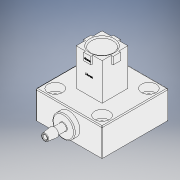
# Autodesk Inventor part: 9mm_ball_holder
Saved by Autodesk Inventor 2019 (Build 230136000, 136)
## iProperties
Created: 2019-03-11
Part Number: 9mm_ball_holder
Material: ABS Plastic
Document SubType Name: Modeling
Designer: Wilson Lab
Density: 1.06 g/cm^3
Appearance: Smooth - White
Author: Wilson Lab
Autodesk Inventor part; units mm, degrees
ref_plane "YZ Plane" through (0, 0, 0) normal (1, 0, 0) x (0, 1, 0)
ref_plane "XZ Plane" through (0, 0, 0) normal (0, 1, 0) x (-1, 0, 0)
ref_plane "XY Plane" through (0, 0, 0) normal (0, 0, 1) x (1, 0, 0)
sketch "Sketch1" plane through (0, 0, 0) normal (0, 0, 1) x (1, 0, 0)
  line L0 (0, 0) -> (-7, 0) construction
  line L1 (-7, 0) -> (-7, 20) construction
  line L2 (-7, 20) -> (0, 20) construction
  line L3 (0, 20) -> (0, 0) construction
  circle A0 centre (0, 20.35) radius 6 construction
  line L4 (-7, 20) -> (-6.6598, 20)
  line L5 (-0.75, 13.7688) -> (-0.75, 0)
  arc A1 (-5.9198, 19.3722) -> (-1.3333, 14.5) centre (0, 20.35) ccw
  arc A2 (-0.75, 13.7688) -> (-1.3333, 14.5) centre (-1.5, 13.7688) ccw
  arc A3 (-5.9198, 19.3722) -> (-6.6598, 20) centre (-6.6598, 19.25) ccw
  line L6 (-7, 20) -> (-7, 0)
  line L7 (-7, 0) -> (-0.75, 0)
  point P0 (-5.9898, 20)
  point P1 (-0.75, 14.3971)
  dimension "d0" = 7
  dimension "d1" = 20
  dimension "d5" = 12
  dimension "d6" = 0.35
  dimension "d7" = 0.75
  dimension "d8" = 0.75
  dimension "d9" = 0.75
  dimension "d132" = 1.0102
  constraints: 18 end point, 10 point on circle, 5 point on line, 4 centre point, 4 tangent, 3 perpendicular, 2 parallel, 1 collinear, 1 concentric, 1 horizontal
  measures "d0" distance between parallel lines of L3 L1
  measures "d1" distance between parallel lines of L0 L2
  measures "d5" diameter of A0
  measures "d6" distance of A0.centre L2.end
  measures "d7" distance between parallel lines of L3 L5
  measures "d8" radius of A2
  measures "d9" radius of A3
  measures "d132" distance of A0.start L1.end
revolve "Revolution1" add sketch "Sketch1" angle 360 about axis through (0, 20, 0) along (0, -1, 0)
ref_plane "Work Plane1" through (0, 20, 0) normal (0, 1, 0) x (1, 0, 0)
sketch "Sketch2" plane through (0, 20, 0) normal (0, 1, 0) x (1, 0, 0)
  circle A0 centre (0, 0) radius 7 projected
  circle A1 centre (0, 0) radius 7 construction
  line L0 (-7, -7) -> (7, -7)
  line L1 (7, -7) -> (7, 7)
  line L2 (7, 7) -> (-7, 7)
  line L3 (-7, 7) -> (-7, -7)
  circle A2 centre (0, 0) radius 1.3333 projected
  line L4 (-7, -7) -> (7, 7) construction
  line L5 (7, -7) -> (-7, 7) construction
  point P0 (0, 0)
  dimension "d124" = 0
  constraints: 12 end point, 2 midpoint, 2 parallel, 2 tangent, 1 centre point, 1 coincident, 1 horizontal, 1 perpendicular
  measures "d124" distance edge to line of A0 L1
extrude "Extrusion1" add sketch "Sketch2" against normal up to surface (20 mm away) contours L1 L0 A0 | A0 L2 L1 | A0 L3 L2 | L0 L3 A0
ref_plane "Work Plane7" through (0, 0, 0) normal (0, -1, 0) x (1, 0, 0)
sketch "Sketch11" plane through (0, 0, 0) normal (0, -1, 0) x (1, 0, 0)
  line L0 (0, 18) -> (0, 0) construction
  line L1 (-18, -18) -> (18, -18)
  line L2 (18, -18) -> (18, 18)
  line L3 (18, 18) -> (-18, 18)
  line L4 (-18, 18) -> (-18, -18)
  line L5 (-18, -18) -> (18, 18) construction
  line L6 (18, -18) -> (-18, 18) construction
  dimension "d60" = 36
  dimension "d61" = 36
  constraints: 14 end point, 3 midpoint, 2 parallel, 1 horizontal, 1 perpendicular
  measures "d60" distance of L1.end L2.end
  measures "d61" distance of L2.end L3.end
extrude "Extrusion6" add sketch "Sketch11" along normal blind 15
sketch "Sketch16" plane through (-18, 0, -18) normal (-1, 0, 0) x (0, 0, 1)
  line L0 (36, 0) -> (0, 0) construction
  line L1 (0, 0) -> (0, -15) construction
  line L2 (36, -15) -> (0, -15) construction
  line L3 (36, 0) -> (36, -15) construction
  line L4 (18.75, 13.7688) -> (18.75, 0) construction
  line L5 (17.25, 13.7688) -> (17.25, 0) construction
  line L6 (18, -7.5) -> (18, 0) construction
  line L7 (36, 0) -> (36, -15) construction
  line L8 (36, 0) -> (36, -7.5) construction
  line L9 (18, -7.5) -> (36, -7.5) construction
  circle A0 centre (18, -7.5) radius 4.225
  dimension "d64" = 8.45
  constraints: 6 end point, 1 centre point, 1 coincident, 1 horizontal, 1 midpoint, 1 vertical
  measures "d64" diameter of A0
extrude "Extrusion7" cut sketch "Sketch16" against normal blind 32.7
sketch "Sketch17" plane through (0, 0, 0) normal (0, -1, 0) x (1, 0, 0)
  circle A0 centre (0, 0) radius 0.75 projected
  point P0 (0, 0)
ref_plane "Work Plane8" through (-18, 0, 0) normal (0, 0, 1) x (1, 0, 0)
sketch "Sketch18" plane through (-18, 0, 0) normal (0, 0, 1) x (1, 0, 0)
  line L0 (18, 0) -> (18, -10.576)
  line L1 (0, -11.725) -> (32.7, -11.725) projected
  constraints: 2 end point, 1 vertical
sweep "Sweep3" cut profiles "Sketch17" path "Sketch18" path curves L0
fillet "Fillet1" radius 3 1 edges at (-0.75, -3.275, -0.001)
sketch "Sketch19" plane through (0, 0, 0) normal (0, 1, 0) x (1, 0, 0)
  line L0 (18, -18) -> (-18, -18) construction
  line L1 (18, 18) -> (18, -18) construction
  line L2 (-18, 18) -> (18, 18) construction
  line L3 (-18, -18) -> (-18, 18) construction
  line L4 (-12.7, 12.7) -> (12.7, 12.7) construction
  line L5 (12.7, 12.7) -> (12.7, -12.7) construction
  line L6 (12.7, -12.7) -> (-12.7, -12.7) construction
  line L7 (-12.7, -12.7) -> (-12.7, 12.7) construction
  circle A0 centre (0, 0) radius 1.3333 construction
  line L8 (-12.7, 12.7) -> (12.7, -12.7) construction
  line L9 (12.7, 12.7) -> (-12.7, -12.7) construction
  point P0 (0, 0)
  dimension "d70" = 25.4
  dimension "d71" = 25.4
  constraints: 12 end point, 4 coincident, 2 midpoint, 2 parallel, 1 horizontal, 1 perpendicular
  measures "d70" distance of L4.end L5.end
  measures "d71" distance of L5.end L6.end
hole "Hole3" at (12.7, 0, -12.7) at (12.7, 0, 12.7) at (-12.7, 0, 12.7) at (-12.7, 0, -12.7) direction (0, -1, 0) diameter 4.496 end through all counterbore diameter 7.938 counterbore depth 4.166
sketch "Sketch21" plane through (-18, 0, 0) normal (0, 0, 1) x (1, 0, 0)
  line L0 (0, -11.725) -> (0, -3.275) construction
  line L1 (0, 0) -> (0, -15) construction
  line L2 (0, -7.5) -> (-3, -7.5)
  line L3 (-3, -9.6296) -> (-3, -13.5)
  line L4 (-3, -13.5) -> (0, -13.5)
  line L5 (0, -13.5) -> (0, -7.5) construction
  line L6 (-3.25, -9.3796) -> (-8, -9.3796)
  arc A0 (-3, -9.6296) -> (-3.25, -9.3796) centre (-3.25, -9.6296) ccw
  line L7 (-8, -9.3796) -> (-8, -9.913)
  line L8 (-8, -9.913) -> (-12.8561, -9.4031)
  line L9 (-8, -9.3796) -> (-13.08, -9.3796) construction
  line L10 (-12.83, -8.65) -> (0, -8.65)
  line L11 (-13.08, -8.9) -> (-13.08, -9.1545)
  arc A1 (-12.83, -8.65) -> (-13.08, -8.9) centre (-12.83, -8.9) ccw
  arc A2 (-13.08, -9.1545) -> (-12.8561, -9.4031) centre (-12.83, -9.1545) ccw
  line L12 (0, -8.65) -> (0, -13.5)
  point P0 (18, 0)
  point P1 (-3, -9.3796)
  dimension "d79" = 3
  dimension "d80" = 6
  dimension "d81" = 5
  dimension "d82" = 1.8796
  dimension "d83" = 0.25
  dimension "d84" = 2.413
  dimension "d85" = 5.08
  dimension "d86" = 1.15
  dimension "d87" = 0.25
  dimension "d88" = 0.25
  constraints: 22 end point, 6 point on circle, 6 point on line, 6 tangent, 3 centre point, 3 horizontal, 2 parallel, 2 perpendicular, 2 vertical, 1 collinear, 1 midpoint
  measures "d79" distance of L3.end L4.end
  measures "d80" distance between parallel lines of L2 L4
  measures "d81" distance of point (-3, -9.38) L6.end
  measures "d82" distance between parallel lines of L2 L6
  measures "d83" radius of A0
  measures "d84" distance from line of L2 L7.end
  measures "d85" horizontal distance of L7.end L9.end
  measures "d86" distance between parallel lines of L10 L2
  measures "d87" radius of A1
  measures "d88" radius of A2
revolve "Revolution2" add sketch "Sketch21" angle 360 about axis through (-18, -7.5, 0) along (-1, 0, 0)
fillet "Fillet2" radius 0.5 9 edges at (-21, -1.5, 0) (0, 0, -18) (-18, 0, 0) (0, 0, 18) (18, 0, 0) (18, -7.5, 18) (-18, -7.5, 18) (-18, -7.5, -18) (18, -7.5, -18)
sketch "Sketch28" plane through (-7, 20, -7) normal (-1, 0, 0) x (0, 0, 1)
  line L0 (0, -20) -> (14, -20) construction
  line L1 (14, 0) -> (14, -20) construction
  line L2 (0, 0) -> (14, 0) construction
  line L3 (0, 0) -> (0, -20) construction
  line L4 (5, -4) -> (9, -4)
  line L5 (9, -4) -> (9, 0)
  line L6 (9, 0) -> (5, 0)
  line L7 (5, 0) -> (5, -4)
  line L8 (5, -2) -> (0, -2) construction
  line L9 (9, -2) -> (14, -2) construction
  point P0 (7, -20)
  dimension "d125" = 0
  dimension "d126" = 4
  constraints: 12 end point, 3 point on line, 2 equal length, 2 midpoint, 2 parallel, 2 perpendicular, 1 horizontal
  measures "d125" distance between parallel lines of L2 L6
  measures "d126" distance of L4.end L5.end
extrude "Extrusion13" add sketch "Sketch28" along normal blind 1
pattern_circular "Circular Pattern1" count 4 over 360 about axis through (0, -10, 0) along (0, 1, 0) of "Extrusion13"
sketch "Sketch30" plane through (-8, 20, -7) normal (-1, 0, 0) x (0, 0, 1)
  line L0 (5, -4) -> (9, -4) construction
  line L1 (9, -4) -> (9, 0) construction
  line L2 (9, 0) -> (5, 0) construction
  line L3 (5, 0) -> (5, -4) construction
  line L4 (5, 0) -> (5, -4) construction
  line L5 (5, -4) -> (5, 0) construction
  line L6 (9, -4) -> (9, 0) construction
  line L7 (9, -4) -> (9, 0) construction
  line L8 (5, -2) -> (9, -2) construction
  line L9 (5, -2) -> (9, -2) construction
  line L10 (9, -2) -> (9, -3.0047) construction
  line L11 (9, -3.0047) -> (5, -3.0047) construction
  line L12 (5, -3.0047) -> (5, -2) construction
  spline S0 degree 2 poles (6.0864, -2.7146) (6.0864, -2.754) (6.0704, -2.7944) (6.0563, -2.7944) knots 0 0 0 1 2 2 2
  line L13 (6.0563, -2.7944) -> (5.9681, -2.7944)
  line L14 (5.9681, -2.7944) -> (5.9681, -2.9737)
  spline S1 degree 2 poles (5.9681, -2.9737) (5.9681, -2.9812) (5.9587, -2.9934) (5.9362, -3.0009) (5.8986, -3.0047) (5.8695, -3.0047) knots 0 0 0 1 2 3 4 4 4
  spline S2 degree 2 poles (5.8695, -3.0047) (5.8423, -3.0047) (5.8047, -3.0009) (5.7822, -2.9934) (5.7737, -2.9812) (5.7737, -2.9737) knots 0 0 0 1 2 3 4 4 4
  line L15 (5.7737, -2.9737) -> (5.7737, -2.7944)
  line L16 (5.7737, -2.7944) -> (5.3925, -2.7944)
  spline S3 degree 2 poles (5.3925, -2.7944) (5.3812, -2.7944) (5.3643, -2.7887) (5.3531, -2.77) (5.3474, -2.7333) (5.3474, -2.7033) knots 0 0 0 1 2 3 4 4 4
  spline S4 degree 2 poles (5.3474, -2.7033) (5.3474, -2.6789) (5.3493, -2.6432) (5.3549, -2.6131) (5.3653, -2.5878) (5.3728, -2.5728) knots 0 0 0 1 2 3 4 4 4
  line L17 (5.3728, -2.5728) -> (5.6826, -2.0272)
  spline S5 degree 2 poles (5.6826, -2.0272) (5.6864, -2.0197) (5.7052, -2.0103) (5.738, -2.0028) (5.7887, -2) (5.8254, -2) knots 0 0 0 1 2 3 4 4 4
  spline S6 degree 2 poles (5.8254, -2) (5.8648, -2) (5.9192, -2.0038) (5.9531, -2.0122) (5.9681, -2.0244) (5.9681, -2.0329) knots 0 0 0 1 2 3 4 4 4
  line L18 (5.9681, -2.0329) -> (5.9681, -2.6329)
  line L19 (5.9681, -2.6329) -> (6.0563, -2.6329)
  spline S7 degree 2 poles (6.0563, -2.6329) (6.0685, -2.6329) (6.0864, -2.6704) (6.0864, -2.7146) knots 0 0 0 1 2 2 2
  line L20 (5.7737, -2.1746) -> (5.7718, -2.1746)
  line L21 (5.7718, -2.1746) -> (5.5089, -2.6329)
  line L22 (5.5089, -2.6329) -> (5.7737, -2.6329)
  line L23 (5.7737, -2.6329) -> (5.7737, -2.1746)
  spline S8 degree 2 poles (7.3061, -2.9737) (7.3061, -2.9812) (7.2967, -2.9934) (7.2751, -3.0009) (7.2385, -3.0047) (7.2094, -3.0047) knots 0 0 0 1 2 3 4 4 4
  spline S9 degree 2 poles (7.2094, -3.0047) (7.1803, -3.0047) (7.1437, -3.0009) (7.1211, -2.9934) (7.1127, -2.9812) (7.1127, -2.9737) knots 0 0 0 1 2 3 4 4 4
  line L24 (7.1127, -2.9737) -> (7.1127, -2.5671)
  spline S10 degree 2 poles (7.1127, -2.5671) (7.1127, -2.5324) (7.0995, -2.4751) (7.0732, -2.4347) (7.0319, -2.4122) (7.0038, -2.4122) knots 0 0 0 1 2 3 4 4 4
  spline S11 degree 2 poles (7.0038, -2.4122) (6.969, -2.4122) (6.8986, -2.4657) (6.8573, -2.5174) knots 0 0 0 1 2 2 2
  line L25 (6.8573, -2.5174) -> (6.8573, -2.9737)
  spline S12 degree 2 poles (6.8573, -2.9737) (6.8573, -2.9812) (6.8479, -2.9934) (6.8254, -3.0009) (6.7887, -3.0047) (6.7606, -3.0047) knots 0 0 0 1 2 3 4 4 4
  spline S13 degree 2 poles (6.7606, -3.0047) (6.7324, -3.0047) (6.6958, -3.0009) (6.6732, -2.9934) (6.6638, -2.9812) (6.6638, -2.9737) knots 0 0 0 1 2 3 4 4 4
  line L26 (6.6638, -2.9737) -> (6.6638, -2.5671)
  spline S14 degree 2 poles (6.6638, -2.5671) (6.6638, -2.5324) (6.6507, -2.4751) (6.6244, -2.4347) (6.5831, -2.4122) (6.5549, -2.4122) knots 0 0 0 1 2 3 4 4 4
  spline S15 degree 2 poles (6.5549, -2.4122) (6.5192, -2.4122) (6.4488, -2.4657) (6.4075, -2.5174) knots 0 0 0 1 2 2 2
  line L27 (6.4075, -2.5174) -> (6.4075, -2.9737)
  spline S16 degree 2 poles (6.4075, -2.9737) (6.4075, -2.9812) (6.3981, -2.9934) (6.3756, -3.0009) (6.339, -3.0047) (6.3108, -3.0047) knots 0 0 0 1 2 3 4 4 4
  spline S17 degree 2 poles (6.3108, -3.0047) (6.2826, -3.0047) (6.246, -3.0009) (6.2235, -2.9934) (6.2141, -2.9812) (6.2141, -2.9737) knots 0 0 0 1 2 3 4 4 4
  line L28 (6.2141, -2.9737) -> (6.2141, -2.2883)
  spline S18 degree 2 poles (6.2141, -2.2883) (6.2141, -2.2808) (6.2216, -2.2685) (6.2413, -2.261) (6.2732, -2.2573) (6.2967, -2.2573) knots 0 0 0 1 2 3 4 4 4
  spline S19 degree 2 poles (6.2967, -2.2573) (6.3211, -2.2573) (6.354, -2.261) (6.3718, -2.2685) (6.3793, -2.2808) (6.3793, -2.2883) knots 0 0 0 1 2 3 4 4 4
  line L29 (6.3793, -2.2883) -> (6.3793, -2.3671)
  spline S20 degree 2 poles (6.3793, -2.3671) (6.4366, -2.3061) (6.5493, -2.2441) (6.6113, -2.2441) knots 0 0 0 1 2 2 2
  spline S21 degree 2 poles (6.6113, -2.2441) (6.6535, -2.2441) (6.7211, -2.262) (6.7746, -2.2948) (6.8131, -2.3408) (6.8263, -2.37) knots 0 0 0 1 2 3 4 4 4
  spline S22 degree 2 poles (6.8263, -2.37) (6.8573, -2.3362) (6.9164, -2.2892) (6.9737, -2.2592) (7.0319, -2.2441) (7.062, -2.2441) knots 0 0 0 1 2 3 4 4 4
  spline S23 degree 2 poles (7.062, -2.2441) (7.1305, -2.2441) (7.2235, -2.2901) (7.2817, -2.369) (7.3061, -2.4761) (7.3061, -2.5352) knots 0 0 0 1 2 3 4 4 4
  line L30 (7.3061, -2.5352) -> (7.3061, -2.9737)
  spline S24 degree 2 poles (8.5878, -2.9737) (8.5878, -2.9812) (8.5784, -2.9934) (8.5568, -3.0009) (8.5202, -3.0047) (8.4911, -3.0047) knots 0 0 0 1 2 3 4 4 4
  spline S25 degree 2 poles (8.4911, -3.0047) (8.462, -3.0047) (8.4254, -3.0009) (8.4028, -2.9934) (8.3944, -2.9812) (8.3944, -2.9737) knots 0 0 0 1 2 3 4 4 4
  line L31 (8.3944, -2.9737) -> (8.3944, -2.5671)
  spline S26 degree 2 poles (8.3944, -2.5671) (8.3944, -2.5324) (8.3812, -2.4751) (8.3549, -2.4347) (8.3136, -2.4122) (8.2854, -2.4122) knots 0 0 0 1 2 3 4 4 4
  spline S27 degree 2 poles (8.2854, -2.4122) (8.2507, -2.4122) (8.1803, -2.4657) (8.139, -2.5174) knots 0 0 0 1 2 2 2
  line L32 (8.139, -2.5174) -> (8.139, -2.9737)
  spline S28 degree 2 poles (8.139, -2.9737) (8.139, -2.9812) (8.1296, -2.9934) (8.107, -3.0009) (8.0704, -3.0047) (8.0423, -3.0047) knots 0 0 0 1 2 3 4 4 4
  spline S29 degree 2 poles (8.0423, -3.0047) (8.0141, -3.0047) (7.9775, -3.0009) (7.9549, -2.9934) (7.9455, -2.9812) (7.9455, -2.9737) knots 0 0 0 1 2 3 4 4 4
  line L33 (7.9455, -2.9737) -> (7.9455, -2.5671)
  spline S30 degree 2 poles (7.9455, -2.5671) (7.9455, -2.5324) (7.9324, -2.4751) (7.9061, -2.4347) (7.8648, -2.4122) (7.8366, -2.4122) knots 0 0 0 1 2 3 4 4 4
  spline S31 degree 2 poles (7.8366, -2.4122) (7.8009, -2.4122) (7.7305, -2.4657) (7.6892, -2.5174) knots 0 0 0 1 2 2 2
  line L34 (7.6892, -2.5174) -> (7.6892, -2.9737)
  spline S32 degree 2 poles (7.6892, -2.9737) (7.6892, -2.9812) (7.6798, -2.9934) (7.6573, -3.0009) (7.6207, -3.0047) (7.5925, -3.0047) knots 0 0 0 1 2 3 4 4 4
  spline S33 degree 2 poles (7.5925, -3.0047) (7.5643, -3.0047) (7.5277, -3.0009) (7.5052, -2.9934) (7.4958, -2.9812) (7.4958, -2.9737) knots 0 0 0 1 2 3 4 4 4
  line L35 (7.4958, -2.9737) -> (7.4958, -2.2883)
  spline S34 degree 2 poles (7.4958, -2.2883) (7.4958, -2.2808) (7.5033, -2.2685) (7.523, -2.261) (7.5549, -2.2573) (7.5784, -2.2573) knots 0 0 0 1 2 3 4 4 4
  spline S35 degree 2 poles (7.5784, -2.2573) (7.6028, -2.2573) (7.6357, -2.261) (7.6535, -2.2685) (7.661, -2.2808) (7.661, -2.2883) knots 0 0 0 1 2 3 4 4 4
  line L36 (7.661, -2.2883) -> (7.661, -2.3671)
  spline S36 degree 2 poles (7.661, -2.3671) (7.7183, -2.3061) (7.831, -2.2441) (7.893, -2.2441) knots 0 0 0 1 2 2 2
  spline S37 degree 2 poles (7.893, -2.2441) (7.9352, -2.2441) (8.0028, -2.262) (8.0563, -2.2948) (8.0948, -2.3408) (8.108, -2.37) knots 0 0 0 1 2 3 4 4 4
  spline S38 degree 2 poles (8.108, -2.37) (8.139, -2.3362) (8.1981, -2.2892) (8.2554, -2.2592) (8.3136, -2.2441) (8.3437, -2.2441) knots 0 0 0 1 2 3 4 4 4
  spline S39 degree 2 poles (8.3437, -2.2441) (8.4122, -2.2441) (8.5052, -2.2901) (8.5634, -2.369) (8.5878, -2.4761) (8.5878, -2.5352) knots 0 0 0 1 2 3 4 4 4
  line L37 (8.5878, -2.5352) -> (8.5878, -2.9737)
  point P0 (7, -20)
  constraints: 6 end point, 4 midpoint, 2 coincident, 2 collinear, 2 other
extrude "Extrusion14" cut sketch "Sketch30" against normal blind 0.5
sketch "Sketch31" plane through (-7, 0, -7) normal (-1, 0, 0) x (0, 0, 1)
  line L0 (9, 20) -> (9, 16) construction
  line L1 (9, 16) -> (5, 16) construction
  line L2 (5, 16) -> (5, 20) construction
  line L3 (0, 20) -> (5, 20) construction
  line L4 (0, 20) -> (0, 0) construction
  line L5 (0, 0) -> (14, 0) construction
  line L6 (14, 20) -> (14, 0) construction
  line L7 (9, 20) -> (14, 20) construction
  line L8 (14, 20) -> (14, 0) construction
  line L9 (14, 20) -> (14, 0) construction
  line L10 (5, 20) -> (0, 20) construction
  line L11 (0, 20) -> (0, 0) construction
  line L12 (0, 10) -> (14, 10) construction
  line L13 (0, 10) -> (14, 10) construction
  line L14 (14, 10) -> (14, 7.8663) construction
  line L15 (14, 7.8663) -> (0, 7.8663) construction
  line L16 (0, 7.8663) -> (0, 10) construction
  spline S0 degree 2 poles (5.6469, 9.0742) (5.6469, 9.0526) (5.6423, 9.0225) (5.6338, 9.0047) (5.6235, 8.9972) (5.616, 8.9972) knots 0 0 0 1 2 3 4 4 4
  line L17 (5.616, 8.9972) -> (5.0667, 8.9972)
  spline S1 degree 2 poles (5.0667, 8.9972) (5.0601, 8.9972) (5.0498, 9.0047) (5.0413, 9.0225) (5.0366, 9.0526) (5.0366, 9.0742) knots 0 0 0 1 2 3 4 4 4
  spline S2 degree 2 poles (5.0366, 9.0742) (5.0366, 9.0958) (5.0404, 9.1258) (5.0488, 9.1446) (5.0601, 9.1531) (5.0667, 9.1531) knots 0 0 0 1 2 3 4 4 4
  line L18 (5.0667, 9.1531) -> (5.2516, 9.1531)
  line L19 (5.2516, 9.1531) -> (5.2516, 9.8019)
  line L20 (5.2516, 9.8019) -> (5.0911, 9.7136)
  spline S3 degree 2 poles (5.0911, 9.7136) (5.0742, 9.7052) (5.0516, 9.7014) (5.0385, 9.7146) (5.0338, 9.7465) (5.0338, 9.7756) knots 0 0 0 1 2 3 4 4 4
  spline S4 degree 2 poles (5.0338, 9.7756) (5.0338, 9.7944) (5.0357, 9.8178) (5.0413, 9.8347) (5.0526, 9.846) (5.062, 9.8516) knots 0 0 0 1 2 3 4 4 4
  line L21 (5.062, 9.8516) -> (5.2751, 9.9897)
  spline S5 degree 2 poles (5.2751, 9.9897) (5.2798, 9.9934) (5.2911, 9.9972) (5.3099, 9.9991) (5.3399, 10) (5.3634, 10) knots 0 0 0 1 2 3 4 4 4
  spline S6 degree 2 poles (5.3634, 10) (5.3925, 10) (5.4291, 9.9981) (5.4469, 9.9925) (5.4535, 9.9831) (5.4535, 9.9765) knots 0 0 0 1 2 3 4 4 4
  line L22 (5.4535, 9.9765) -> (5.4535, 9.1531)
  line L23 (5.4535, 9.1531) -> (5.616, 9.1531)
  spline S7 degree 2 poles (5.616, 9.1531) (5.6235, 9.1531) (5.6347, 9.1446) (5.6432, 9.1258) (5.6469, 9.0958) (5.6469, 9.0742) knots 0 0 0 1 2 3 4 4 4
  spline S8 degree 2 poles (6.4854, 9.2826) (6.4854, 9.2432) (6.4695, 9.2028) (6.4554, 9.2028) knots 0 0 0 1 2 2 2
  line L24 (6.4554, 9.2028) -> (6.3671, 9.2028)
  line L25 (6.3671, 9.2028) -> (6.3671, 9.0235)
  spline S9 degree 2 poles (6.3671, 9.0235) (6.3671, 9.016) (6.3577, 9.0038) (6.3352, 8.9962) (6.2977, 8.9925) (6.2685, 8.9925) knots 0 0 0 1 2 3 4 4 4
  spline S10 degree 2 poles (6.2685, 8.9925) (6.2413, 8.9925) (6.2038, 8.9962) (6.1812, 9.0038) (6.1728, 9.016) (6.1728, 9.0235) knots 0 0 0 1 2 3 4 4 4
  line L26 (6.1728, 9.0235) -> (6.1728, 9.2028)
  line L27 (6.1728, 9.2028) -> (5.7915, 9.2028)
  spline S11 degree 2 poles (5.7915, 9.2028) (5.7803, 9.2028) (5.7634, 9.2085) (5.7521, 9.2272) (5.7465, 9.2638) (5.7465, 9.2939) knots 0 0 0 1 2 3 4 4 4
  spline S12 degree 2 poles (5.7465, 9.2939) (5.7465, 9.3183) (5.7484, 9.354) (5.754, 9.384) (5.7643, 9.4094) (5.7718, 9.4244) knots 0 0 0 1 2 3 4 4 4
  line L28 (5.7718, 9.4244) -> (6.0817, 9.97)
  spline S13 degree 2 poles (6.0817, 9.97) (6.0854, 9.9775) (6.1042, 9.9869) (6.1371, 9.9944) (6.1878, 9.9972) (6.2244, 9.9972) knots 0 0 0 1 2 3 4 4 4
  spline S14 degree 2 poles (6.2244, 9.9972) (6.2638, 9.9972) (6.3183, 9.9934) (6.3521, 9.985) (6.3671, 9.9728) (6.3671, 9.9643) knots 0 0 0 1 2 3 4 4 4
  line L29 (6.3671, 9.9643) -> (6.3671, 9.3643)
  line L30 (6.3671, 9.3643) -> (6.4554, 9.3643)
  spline S15 degree 2 poles (6.4554, 9.3643) (6.4676, 9.3643) (6.4854, 9.3268) (6.4854, 9.2826) knots 0 0 0 1 2 2 2
  line L31 (6.1728, 9.8225) -> (6.1709, 9.8225)
  line L32 (6.1709, 9.8225) -> (5.908, 9.3643)
  line L33 (5.908, 9.3643) -> (6.1728, 9.3643)
  line L34 (6.1728, 9.3643) -> (6.1728, 9.8225)
  spline S16 degree 2 poles (7.7052, 9.0235) (7.7052, 9.016) (7.6958, 9.0038) (7.6742, 8.9962) (7.6376, 8.9925) (7.6085, 8.9925) knots 0 0 0 1 2 3 4 4 4
  spline S17 degree 2 poles (7.6085, 8.9925) (7.5793, 8.9925) (7.5427, 8.9962) (7.5202, 9.0038) (7.5117, 9.016) (7.5117, 9.0235) knots 0 0 0 1 2 3 4 4 4
  line L35 (7.5117, 9.0235) -> (7.5117, 9.43)
  spline S18 degree 2 poles (7.5117, 9.43) (7.5117, 9.4648) (7.4986, 9.5221) (7.4723, 9.5624) (7.431, 9.585) (7.4028, 9.585) knots 0 0 0 1 2 3 4 4 4
  spline S19 degree 2 poles (7.4028, 9.585) (7.3681, 9.585) (7.2977, 9.5315) (7.2563, 9.4798) knots 0 0 0 1 2 2 2
  line L36 (7.2563, 9.4798) -> (7.2563, 9.0235)
  spline S20 degree 2 poles (7.2563, 9.0235) (7.2563, 9.016) (7.2469, 9.0038) (7.2244, 8.9962) (7.1878, 8.9925) (7.1596, 8.9925) knots 0 0 0 1 2 3 4 4 4
  spline S21 degree 2 poles (7.1596, 8.9925) (7.1315, 8.9925) (7.0948, 8.9962) (7.0723, 9.0038) (7.0629, 9.016) (7.0629, 9.0235) knots 0 0 0 1 2 3 4 4 4
  line L37 (7.0629, 9.0235) -> (7.0629, 9.43)
  spline S22 degree 2 poles (7.0629, 9.43) (7.0629, 9.4648) (7.0498, 9.5221) (7.0235, 9.5624) (6.9822, 9.585) (6.954, 9.585) knots 0 0 0 1 2 3 4 4 4
  spline S23 degree 2 poles (6.954, 9.585) (6.9183, 9.585) (6.8479, 9.5315) (6.8066, 9.4798) knots 0 0 0 1 2 2 2
  line L38 (6.8066, 9.4798) -> (6.8066, 9.0235)
  spline S24 degree 2 poles (6.8066, 9.0235) (6.8066, 9.016) (6.7972, 9.0038) (6.7746, 8.9962) (6.738, 8.9925) (6.7099, 8.9925) knots 0 0 0 1 2 3 4 4 4
  spline S25 degree 2 poles (6.7099, 8.9925) (6.6817, 8.9925) (6.6451, 8.9962) (6.6225, 9.0038) (6.6131, 9.016) (6.6131, 9.0235) knots 0 0 0 1 2 3 4 4 4
  line L39 (6.6131, 9.0235) -> (6.6131, 9.7089)
  spline S26 degree 2 poles (6.6131, 9.7089) (6.6131, 9.7164) (6.6207, 9.7286) (6.6404, 9.7362) (6.6723, 9.7399) (6.6958, 9.7399) knots 0 0 0 1 2 3 4 4 4
  spline S27 degree 2 poles (6.6958, 9.7399) (6.7202, 9.7399) (6.7531, 9.7362) (6.7709, 9.7286) (6.7784, 9.7164) (6.7784, 9.7089) knots 0 0 0 1 2 3 4 4 4
  line L40 (6.7784, 9.7089) -> (6.7784, 9.63)
  spline S28 degree 2 poles (6.7784, 9.63) (6.8357, 9.6911) (6.9484, 9.7531) (7.0103, 9.7531) knots 0 0 0 1 2 2 2
  spline S29 degree 2 poles (7.0103, 9.7531) (7.0526, 9.7531) (7.1202, 9.7352) (7.1737, 9.7023) (7.2122, 9.6563) (7.2254, 9.6272) knots 0 0 0 1 2 3 4 4 4
  spline S30 degree 2 poles (7.2254, 9.6272) (7.2563, 9.661) (7.3155, 9.708) (7.3728, 9.738) (7.431, 9.7531) (7.461, 9.7531) knots 0 0 0 1 2 3 4 4 4
  spline S31 degree 2 poles (7.461, 9.7531) (7.5296, 9.7531) (7.6225, 9.707) (7.6808, 9.6282) (7.7052, 9.5211) (7.7052, 9.462) knots 0 0 0 1 2 3 4 4 4
  line L41 (7.7052, 9.462) -> (7.7052, 9.0235)
  spline S32 degree 2 poles (8.9869, 9.0235) (8.9869, 9.016) (8.9775, 9.0038) (8.9559, 8.9962) (8.9192, 8.9925) (8.8901, 8.9925) knots 0 0 0 1 2 3 4 4 4
  spline S33 degree 2 poles (8.8901, 8.9925) (8.861, 8.9925) (8.8244, 8.9962) (8.8019, 9.0038) (8.7934, 9.016) (8.7934, 9.0235) knots 0 0 0 1 2 3 4 4 4
  line L42 (8.7934, 9.0235) -> (8.7934, 9.43)
  spline S34 degree 2 poles (8.7934, 9.43) (8.7934, 9.4648) (8.7803, 9.5221) (8.754, 9.5624) (8.7127, 9.585) (8.6845, 9.585) knots 0 0 0 1 2 3 4 4 4
  spline S35 degree 2 poles (8.6845, 9.585) (8.6498, 9.585) (8.5793, 9.5315) (8.538, 9.4798) knots 0 0 0 1 2 2 2
  line L43 (8.538, 9.4798) -> (8.538, 9.0235)
  spline S36 degree 2 poles (8.538, 9.0235) (8.538, 9.016) (8.5286, 9.0038) (8.5061, 8.9962) (8.4695, 8.9925) (8.4413, 8.9925) knots 0 0 0 1 2 3 4 4 4
  spline S37 degree 2 poles (8.4413, 8.9925) (8.4131, 8.9925) (8.3765, 8.9962) (8.354, 9.0038) (8.3446, 9.016) (8.3446, 9.0235) knots 0 0 0 1 2 3 4 4 4
  line L44 (8.3446, 9.0235) -> (8.3446, 9.43)
  spline S38 degree 2 poles (8.3446, 9.43) (8.3446, 9.4648) (8.3315, 9.5221) (8.3052, 9.5624) (8.2638, 9.585) (8.2357, 9.585) knots 0 0 0 1 2 3 4 4 4
  spline S39 degree 2 poles (8.2357, 9.585) (8.2, 9.585) (8.1296, 9.5315) (8.0883, 9.4798) knots 0 0 0 1 2 2 2
  line L45 (8.0883, 9.4798) -> (8.0883, 9.0235)
  spline S40 degree 2 poles (8.0883, 9.0235) (8.0883, 9.016) (8.0789, 9.0038) (8.0563, 8.9962) (8.0197, 8.9925) (7.9915, 8.9925) knots 0 0 0 1 2 3 4 4 4
  spline S41 degree 2 poles (7.9915, 8.9925) (7.9634, 8.9925) (7.9268, 8.9962) (7.9042, 9.0038) (7.8948, 9.016) (7.8948, 9.0235) knots 0 0 0 1 2 3 4 4 4
  line L46 (7.8948, 9.0235) -> (7.8948, 9.7089)
  spline S42 degree 2 poles (7.8948, 9.7089) (7.8948, 9.7164) (7.9023, 9.7286) (7.9221, 9.7362) (7.954, 9.7399) (7.9775, 9.7399) knots 0 0 0 1 2 3 4 4 4
  spline S43 degree 2 poles (7.9775, 9.7399) (8.0019, 9.7399) (8.0347, 9.7362) (8.0526, 9.7286) (8.0601, 9.7164) (8.0601, 9.7089) knots 0 0 0 1 2 3 4 4 4
  line L47 (8.0601, 9.7089) -> (8.0601, 9.63)
  spline S44 degree 2 poles (8.0601, 9.63) (8.1174, 9.6911) (8.23, 9.7531) (8.292, 9.7531) knots 0 0 0 1 2 2 2
  spline S45 degree 2 poles (8.292, 9.7531) (8.3343, 9.7531) (8.4019, 9.7352) (8.4554, 9.7023) (8.4939, 9.6563) (8.507, 9.6272) knots 0 0 0 1 2 3 4 4 4
  spline S46 degree 2 poles (8.507, 9.6272) (8.538, 9.661) (8.5972, 9.708) (8.6545, 9.738) (8.7127, 9.7531) (8.7427, 9.7531) knots 0 0 0 1 2 3 4 4 4
  spline S47 degree 2 poles (8.7427, 9.7531) (8.8113, 9.7531) (8.9042, 9.707) (8.9624, 9.6282) (8.9869, 9.5211) (8.9869, 9.462) knots 0 0 0 1 2 3 4 4 4
  line L48 (8.9869, 9.462) -> (8.9869, 9.0235)
  point P0 (7, 0)
  constraints: 6 end point, 4 midpoint, 2 coincident, 2 collinear, 2 other
extrude "Extrusion15" cut sketch "Sketch31" against normal blind 0.5
body "Solid1"
